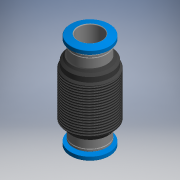
# Autodesk Inventor part: 153160 QSS-10---(part)
Saved by Autodesk Inventor 2017.3 (Build 213256000, 256)
## iProperties
Part Number: 153160 QSS-10---(part)
Material: Generic
Catalog Web Link: www.cadenas.de
Description: QSS_p-Push-in bulkhead connector
Vendor: FESTO
Document SubType Name: Modeling
Designer: partserver
Manufacturer: FESTO
Mass: 37 g
Surface Area: 44.3669 cm^2
Volume: 7.16815 cm^3
Density: 1 g/cm^3
Appearance: PSOLRGB-175-175-175
Category: PARTsolutions
Company: FESTO
Title: 153160 QSS-10---(part)
Author: Cadenas PARTsolutions
Comments: Push-in bulkhead connector
PSOL_IDENT_0: {$CADENAS_DATA\23d-libs\festo\parts\q\qss\parts\qss_p.prj},183 {VTYP=3D},{NB=153160 QSS-10---(part)}
PSOL_IDENT_1: ,{LINA=153160 QSS-10---(part)},{NN=QSS_p},{DATE=12.05.2017 09:34:06},{GEOMDATE=26.04.2016 11:15:02},
PSOL_IDENT_2: {VERSION=},{LINEID=40},{WBVAR=},{WBNUMERIC=}  {NB=153160 QSS-10---(part)},{LINA=153160 QSS-10---(par
PSOL_IDENT_3: t)},{KT=DUMMY},{TNR=153160},{TYP=QSS-10},{D1=10},{NENN=9.000},{D5=M20X1},{D6=18.500},{L1=42.400},{L2=
PSOL_IDENT_4: 21.600},{L3=11.900},{SW=24.000},{T=20.700},{CNSMASSEXACT=0.037},{D5N=20.000},{Z=16.800},{D12=15.600}
NB: 153160 QSS-10---(part)
NN: QSS_p
NT: Push-in bulkhead connector
NBSYN: $TNR. $TYP.---(part)
LINA: 153160 QSS-10---(part)
CATALOG: Festo
TNR: 153160
TYP: QSS-10
D1: 10
NENN: 9
D5: M20X1
D6: 18.5
L1: 42.4
L2: 21.6
L3: 11.9
SW: 24
T: 20.7
CNSMASSEXACT: 0.037
D5N: 20
SUPPLIER: FESTO
ARTICLENO: 153160 QSS-10---(part)
BOMINFO: 153160 QSS-10---(part)
CREATOR: CADENAS GmbH
Autodesk Inventor part; units mm, degrees
ref_plane "YZ Plane" through (0, 0, 0) normal (1, 0, 0) x (0, 1, 0)
ref_plane "XZ Plane" through (0, 0, 0) normal (0, 1, 0) x (-1, 0, 0)
ref_plane "XY Plane" through (0, 0, 0) normal (0, 0, 1) x (1, 0, 0)
sketch "Sketch_1" plane through (0, 0, 0) normal (1, 0, 0) x (0, 1, 0)
  line L0 (0, 0) -> (0, 42.4)
  line L1 (0, 42.4) -> (5.3, 42.4)
  line L2 (5.3, 42.4) -> (8.2347, 41.8825)
  arc A0 (8.4, 41.6856) -> (8.2347, 41.8825) centre (8.2, 41.6856) ccw
  line L3 (8.4, 41.6856) -> (8.4, 40.3)
  line L4 (8.4, 40.3) -> (6, 40.3)
  arc A1 (6, 40.3) -> (5.7, 40) centre (6, 40) ccw
  line L5 (5.7, 40) -> (5.7, 39.3)
  line L6 (5.7, 39.3) -> (7.1, 39.3)
  line L7 (7.1, 39.3) -> (7.2, 39.2)
  line L8 (7.2, 39.2) -> (7.2, 38.4678)
  line L9 (7.2, 38.4678) -> (7, 38.3)
  line L10 (7, 38.3) -> (7.2, 38.1322)
  line L11 (7.2, 38.1322) -> (7.2, 34.4)
  line L12 (7.2, 34.4) -> (7.8, 34.4)
  line L13 (7.8, 34.4) -> (8.3196, 33.5)
  line L14 (8.3196, 33.5) -> (10, 31.8196)
  line L15 (10, 31.8196) -> (10, 12.65)
  line L16 (10, 12.65) -> (9.25, 11.9)
  line L17 (9.25, 11.9) -> (9.25, 9.8304)
  line L18 (9.25, 9.8304) -> (8.3196, 8.9)
  line L19 (8.3196, 8.9) -> (7.8, 8)
  line L20 (7.8, 8) -> (7.2, 8)
  line L21 (7.2, 8) -> (7.2, 4.2678)
  line L22 (7.2, 4.2678) -> (7, 4.1)
  line L23 (7, 4.1) -> (7.2, 3.9322)
  line L24 (7.2, 3.9322) -> (7.2, 3.2)
  line L25 (7.2, 3.2) -> (7.1, 3.1)
  line L26 (7.1, 3.1) -> (5.7, 3.1)
  line L27 (5.7, 3.1) -> (5.7, 2.4)
  arc A2 (5.7, 2.4) -> (6, 2.1) centre (6, 2.4) ccw
  line L28 (6, 2.1) -> (8.4, 2.1)
  line L29 (8.4, 2.1) -> (8.4, 0.7144)
  arc A3 (8.2347, 0.5175) -> (8.4, 0.7144) centre (8.2, 0.7144) ccw
  line L30 (8.2347, 0.5175) -> (5.3, 0)
  line L31 (5.3, 0) -> (0, 0)
  line L32 (0, 0) -> (0, 42.4)
  constraints: 66 end point, 8 point on circle, 4 centre point
revolve "Revolution1" add sketch "Sketch_1" angle 360 about axis through (0, 0, 0) along (0, 0, -1)
thread "Thread1" size "M20x1" class "6g" standard "ISO Metric profile" full length
sketch "Sketch_4" plane through (0, 0, 0) normal (1, 0, 0) x (0, 1, 0)
  line L0 (0, 0) -> (0, 42.4)
  line L1 (0, 42.4) -> (5.3, 42.4)
  arc A0 (5.3, 42.4) -> (5, 42.1) centre (5.3, 42.1) ccw
  line L2 (5, 42.1) -> (5, 21.7)
  line L3 (5, 21.7) -> (4.5, 21.7)
  line L4 (4.5, 21.7) -> (4.5, 20.7)
  line L5 (4.5, 20.7) -> (5, 20.7)
  line L6 (5, 20.7) -> (5, 0.3)
  arc A1 (5, 0.3) -> (5.3, 0) centre (5.3, 0.3) ccw
  line L7 (5.3, 0) -> (0, 0)
  line L8 (0, 0) -> (0, 42.4)
  constraints: 18 end point, 4 point on circle, 2 centre point
revolve "Revolution2" cut sketch "Sketch_4" angle 360 about axis through (0, 0, 0) along (0, 0, -1)
ref_plane "ANBAU_XY" through (0, 0, 0) normal (0, 0, -1) x (1, 0, 0)
ref_plane "ANBAU_YZ" through (0, 0, 0) normal (1, 0, 0) x (0, -1, 0)
ref_plane "ANBAU_ZX" through (0, 0, 0) normal (0, -1, 0) x (0, 0, -1)
ref_plane "IP1_XY" through (0, 0, 32) normal (0, 0, -1) x (1, 0, 0)
ref_plane "IP1_YZ" through (0, 0, 32) normal (1, 0, 0) x (0, -1, 0)
ref_plane "IP1_ZX" through (0, 0, 32) normal (0, -1, 0) x (0, 0, -1)
ref_plane "IP2_XY" through (0, 0, 14.4) normal (0, 0, -1) x (1, 0, 0)
ref_plane "IP2_YZ" through (0, 0, 14.4) normal (1, 0, 0) x (0, -1, 0)
ref_plane "IP2_ZX" through (0, 0, 14.4) normal (0, -1, 0) x (0, 0, -1)
body "Solid1"
